Autodesk Inventor part; units mm, degrees
(part 6 of 7)
  line L4288 (-217.7033, 32.4949) -> (-217.7088, 32.0158)
  line L4289 (-217.7088, 32.0158) -> (-217.7607, 31.5383)
  line L4290 (-217.7607, 31.5383) -> (-217.8407, 31.2539)
  line L4291 (-217.8407, 31.2539) -> (-217.9599, 30.9836)
  line L4292 (-217.9599, 30.9836) -> (-218.06, 30.829)
  line L4293 (-218.06, 30.829) -> (-218.1762, 30.6868)
  line L4294 (-218.1762, 30.6868) -> (-218.3073, 30.5582)
  line L4295 (-218.3073, 30.5582) -> (-218.4521, 30.4446)
  line L4296 (-218.4521, 30.4446) -> (-218.6077, 30.3605)
  line L4297 (-218.6077, 30.3605) -> (-218.7713, 30.295)
  line L4298 (-218.7713, 30.295) -> (-218.9414, 30.2486)
  line L4299 (-218.9414, 30.2486) -> (-219.1162, 30.2219)
  line L4300 (-219.1162, 30.2219) -> (-219.7927, 30.1616)
  line L4301 (-219.7927, 30.1616) -> (-220.4717, 30.1477)
  line L4302 (-220.4717, 30.1477) -> (-225.6943, 30.1477)
  line L4303 (-225.6943, 30.1477) -> (-225.6943, 29.0188)
  line L4304 (-225.6943, 29.0188) -> (-226.8896, 29.0188)
  line L4305 (-226.8896, 29.0188) -> (-226.8896, 30.1477)
  line L4306 (-226.8896, 30.1477) -> (-229.1357, 30.1477)
  line L4307 (-229.1357, 30.1477) -> (-230.0615, 31.675)
  line L4308 (-230.0615, 31.675) -> (-226.8896, 31.675)
  line L4309 (-227.0654, -1.5867) -> (-226.9717, -1.1921)
  line L4310 (-226.9717, -1.1921) -> (-226.8154, -0.7976)
  line L4311 (-226.8154, -0.7976) -> (-226.6006, -0.3953)
  line L4312 (-226.6006, -0.3953) -> (-225.1709, -0.9265)
  line L4313 (-225.1709, -0.9265) -> (-225.3114, -1.1898)
  line L4314 (-225.3114, -1.1898) -> (-225.415, -1.4683)
  line L4315 (-225.415, -1.4683) -> (-225.4805, -1.7581)
  line L4316 (-225.4805, -1.7581) -> (-225.5068, -2.0554)
  line L4317 (-225.5068, -2.0554) -> (-225.4604, -2.423)
  line L4318 (-225.4604, -2.423) -> (-225.3285, -2.7636)
  line L4319 (-225.3285, -2.7636) -> (-225.1187, -3.0626)
  line L4320 (-225.1187, -3.0626) -> (-224.8389, -3.3054)
  line L4321 (-224.8389, -3.3054) -> (-224.6095, -3.4375)
  line L4322 (-224.6095, -3.4375) -> (-224.3623, -3.532)
  line L4323 (-224.3623, -3.532) -> (-223.9212, -3.6468)
  line L4324 (-223.9212, -3.6468) -> (-223.4735, -3.7282)
  line L4325 (-223.4735, -3.7282) -> (-223.0209, -3.7759)
  line L4326 (-223.0209, -3.7759) -> (-222.5654, -3.7898)
  line L4327 (-222.5654, -3.7898) -> (-217.8154, -3.7898)
  line L4328 (-217.8154, -3.7898) -> (-217.8154, -5.325)
  line L4329 (-217.8154, -5.325) -> (-226.8896, -5.325)
  line L4330 (-226.8896, -5.325) -> (-226.8896, -3.9421)
  line L4331 (-226.8896, -3.9421) -> (-225.5146, -3.9421)
  line L4332 (-225.5146, -3.9421) -> (-225.803, -3.7828)
  line L4333 (-225.803, -3.7828) -> (-226.0795, -3.6042)
  line L4334 (-226.0795, -3.6042) -> (-226.343, -3.4071)
  line L4335 (-226.343, -3.4071) -> (-226.5928, -3.1921)
  line L4336 (-226.5928, -3.1921) -> (-226.6972, -3.0847)
  line L4337 (-226.6972, -3.0847) -> (-226.7881, -2.9656)
  line L4338 (-226.7881, -2.9656) -> (-226.921, -2.7383)
  line L4339 (-226.921, -2.7383) -> (-227.0177, -2.495)
  line L4340 (-227.0177, -2.495) -> (-227.0767, -2.2399)
  line L4341 (-227.0767, -2.2399) -> (-227.0967, -1.9773)
  line L4342 (-227.0967, -1.9773) -> (-227.0654, -1.5867)
  line L4343 (-227.0654, 12.9368) -> (-226.9717, 13.3313)
  line L4344 (-226.9717, 13.3313) -> (-226.8154, 13.7297)
  line L4345 (-226.8154, 13.7297) -> (-226.6006, 14.1282)
  line L4346 (-226.6006, 14.1282) -> (-225.1709, 13.6008)
  line L4347 (-225.1709, 13.6008) -> (-225.3106, 13.3372)
  line L4348 (-225.3106, 13.3372) -> (-225.4139, 13.0587)
  line L4349 (-225.4139, 13.0587) -> (-225.4797, 12.769)
  line L4350 (-225.4797, 12.769) -> (-225.5068, 12.4719)
  line L4351 (-225.5068, 12.4719) -> (-225.4616, 12.1038)
  line L4352 (-225.4616, 12.1038) -> (-225.33, 11.763)
  line L4353 (-225.33, 11.763) -> (-225.1197, 11.464)
  line L4354 (-225.1197, 11.464) -> (-224.8389, 11.2219)
  line L4355 (-224.8389, 11.2219) -> (-224.6089, 11.0895)
  line L4356 (-224.6089, 11.0895) -> (-224.3623, 10.9914)
  line L4357 (-224.3623, 10.9914) -> (-223.9213, 10.877)
  line L4358 (-223.9213, 10.877) -> (-223.4735, 10.7964)
  line L4359 (-223.4735, 10.7964) -> (-223.0209, 10.7498)
  line L4360 (-223.0209, 10.7498) -> (-222.5654, 10.7375)
  line L4361 (-222.5654, 10.7375) -> (-217.8154, 10.7375)
  line L4362 (-217.8154, 10.7375) -> (-217.8154, 9.1985)
  line L4363 (-217.8154, 9.1985) -> (-226.8896, 9.1985)
  line L4364 (-226.8896, 9.1985) -> (-226.8896, 10.5813)
  line L4365 (-226.8896, 10.5813) -> (-225.5146, 10.5813)
  line L4366 (-225.5146, 10.5813) -> (-225.8025, 10.7415)
  line L4367 (-225.8025, 10.7415) -> (-226.0787, 10.9203)
  line L4368 (-226.0787, 10.9203) -> (-226.3424, 11.1171)
  line L4369 (-226.3424, 11.1171) -> (-226.5928, 11.3313)
  line L4370 (-226.5928, 11.3313) -> (-226.7777, 11.5469)
  line L4371 (-226.7777, 11.5469) -> (-226.9209, 11.7922)
  line L4372 (-226.9209, 11.7922) -> (-226.9978, 11.972)
  line L4373 (-226.9978, 11.972) -> (-227.0531, 12.1589)
  line L4374 (-227.0531, 12.1589) -> (-227.0862, 12.3509)
  line L4375 (-227.0862, 12.3509) -> (-227.0967, 12.5461)
  line L4376 (-227.0967, 12.5461) -> (-227.0654, 12.9368)
  line L4377 (-225.1982, -44.1804) -> (-225.1982, -37.6687)
  line L4378 (-225.1982, -37.6687) -> (-230.3428, -37.6687)
  line L4379 (-230.3428, -37.6687) -> (-230.3428, -36.0086)
  line L4380 (-230.3428, -36.0086) -> (-217.8154, -36.0086)
  line L4381 (-217.8154, -36.0086) -> (-217.8154, -37.6687)
  line L4382 (-217.8154, -37.6687) -> (-223.7217, -37.6687)
  line L4383 (-223.7217, -37.6687) -> (-223.7217, -44.1804)
  line L4384 (-223.7217, -44.1804) -> (-217.8154, -44.1804)
  line L4385 (-217.8154, -44.1804) -> (-217.8154, -45.8367)
  line L4386 (-217.8154, -45.8367) -> (-230.3428, -45.8367)
  line L4387 (-230.3428, -45.8367) -> (-230.3428, -44.1804)
  line L4388 (-230.3428, -44.1804) -> (-225.1982, -44.1804)
  line L4389 (-221.456, -21.0437) -> (-220.5474, -20.7358)
  line L4390 (-220.5474, -20.7358) -> (-219.6279, -20.4617)
  line L4391 (-219.6279, -20.4617) -> (-220.4966, -20.1929)
  line L4392 (-220.4966, -20.1929) -> (-221.3545, -19.8914)
  line L4393 (-221.3545, -19.8914) -> (-226.8896, -17.8757)
  line L4394 (-226.8896, -17.8757) -> (-226.8896, -16.2937)
  line L4395 (-226.8896, -16.2937) -> (-217.8154, -19.7273)
  line L4396 (-217.8154, -19.7273) -> (-217.8154, -21.1648)
  line L4397 (-217.8154, -21.1648) -> (-226.8896, -24.6179)
  line L4398 (-226.8896, -24.6179) -> (-226.8896, -22.9929)
  line L4399 (-226.8896, -22.9929) -> (-221.456, -21.0437)
  line L4400 (-230.5459, 28.0032) -> (-230.4917, 28.5563)
  line L4401 (-230.4917, 28.5563) -> (-230.4014, 29.1047)
  line L4402 (-230.4014, 29.1047) -> (-229.0615, 28.8743)
  line L4403 (-229.0615, 28.8743) -> (-229.1228, 28.4229)
  line L4404 (-229.1228, 28.4229) -> (-229.1474, 27.968)
  line L4405 (-229.1474, 27.968) -> (-229.1237, 27.6049)
  line L4406 (-229.1237, 27.6049) -> (-229.0303, 27.2532)
  line L4407 (-229.0303, 27.2532) -> (-228.9284, 27.0739)
  line L4408 (-228.9284, 27.0739) -> (-228.7871, 26.9279)
  line L4409 (-228.7871, 26.9279) -> (-228.6141, 26.8216)
  line L4410 (-228.6141, 26.8216) -> (-228.417, 26.761)
  line L4411 (-228.417, 26.761) -> (-228.0735, 26.7027)
  line L4412 (-228.0735, 26.7027) -> (-227.7256, 26.6868)
  line L4413 (-227.7256, 26.6868) -> (-226.8896, 26.6868)
  line L4414 (-226.8896, 26.6868) -> (-226.8896, 28.4563)
  line L4415 (-226.8896, 28.4563) -> (-225.6943, 28.4563)
  line L4416 (-225.6943, 28.4563) -> (-225.6943, 26.6868)
  line L4417 (-225.6943, 26.6868) -> (-217.8154, 26.6868)
  line L4418 (-217.8154, 26.6868) -> (-217.8154, 25.1594)
  line L4419 (-217.8154, 25.1594) -> (-225.6943, 25.1594)
  line L4420 (-225.6943, 25.1594) -> (-225.6943, 23.8)
  line L4421 (-225.6943, 23.8) -> (-226.8896, 23.8)
  line L4422 (-226.8896, 23.8) -> (-226.8896, 25.1594)
  line L4423 (-226.8896, 25.1594) -> (-227.5869, 25.157)
  line L4424 (-227.5869, 25.157) -> (-228.2842, 25.1672)
  line L4425 (-228.2842, 25.1672) -> (-228.6256, 25.1953)
  line L4426 (-228.6256, 25.1953) -> (-228.9639, 25.2493)
  line L4427 (-228.9639, 25.2493) -> (-229.2139, 25.3196)
  line L4428 (-229.2139, 25.3196) -> (-229.499, 25.4524)
  line L4429 (-229.499, 25.4524) -> (-229.7568, 25.6282)
  line L4430 (-229.7568, 25.6282) -> (-229.9834, 25.843)
  line L4431 (-229.9834, 25.843) -> (-230.1395, 26.0379)
  line L4432 (-230.1395, 26.0379) -> (-230.2724, 26.2493)
  line L4433 (-230.2724, 26.2493) -> (-230.3897, 26.5305)
  line L4434 (-230.3897, 26.5305) -> (-230.4754, 26.822)
  line L4435 (-230.4754, 26.822) -> (-230.529, 27.1211)
  line L4436 (-230.529, 27.1211) -> (-230.5498, 27.425)
  line L4437 (-230.5498, 27.425) -> (-230.5575, 27.7142)
  line L4438 (-230.5575, 27.7142) -> (-230.5459, 28.0032)
  line L4439 (-222.2842, 20.5618) -> (-222.123, 19.998)
  line L4440 (-222.123, 19.998) -> (-221.9865, 19.428)
  line L4441 (-221.9865, 19.428) -> (-221.8748, 18.8526)
  line L4442 (-221.8748, 18.8526) -> (-221.7881, 18.2727)
  line L4443 (-221.7881, 18.2727) -> (-221.6865, 17.6488)
  line L4444 (-221.6865, 17.6488) -> (-221.5224, 17.0383)
  line L4445 (-221.5224, 17.0383) -> (-221.4547, 16.8714)
  line L4446 (-221.4547, 16.8714) -> (-221.3669, 16.715)
  line L4447 (-221.3669, 16.715) -> (-221.2602, 16.5708)
  line L4448 (-221.2602, 16.5708) -> (-221.1357, 16.4407)
  line L4449 (-221.1357, 16.4407) -> (-220.9118, 16.2821)
  line L4450 (-220.9118, 16.2821) -> (-220.6683, 16.1747)
  line L4451 (-220.6683, 16.1747) -> (-220.4128, 16.1178)
  line L4452 (-220.4128, 16.1178) -> (-220.1531, 16.111)
  line L4453 (-220.1531, 16.111) -> (-219.8968, 16.1537)
  line L4454 (-219.8968, 16.1537) -> (-219.6517, 16.2453)
  line L4455 (-219.6517, 16.2453) -> (-219.4254, 16.3855)
  line L4456 (-219.4254, 16.3855) -> (-219.2256, 16.5735)
  line L4457 (-219.2256, 16.5735) -> (-219.101, 16.7434)
  line L4458 (-219.101, 16.7434) -> (-219.0001, 16.9273)
  line L4459 (-219.0001, 16.9273) -> (-218.9241, 17.1227)
  line L4460 (-218.9241, 17.1227) -> (-218.874, 17.3274)
  line L4461 (-218.874, 17.3274) -> (-218.8298, 17.6306)
  line L4462 (-218.8298, 17.6306) -> (-218.8154, 17.9368)
  line L4463 (-218.8154, 17.9368) -> (-218.8389, 18.3704)
  line L4464 (-218.8389, 18.3704) -> (-218.9131, 18.7766)
  line L4465 (-218.9131, 18.7766) -> (-219.0342, 19.1594)
  line L4466 (-219.0342, 19.1594) -> (-219.2021, 19.5188)
  line L4467 (-219.2021, 19.5188) -> (-219.417, 19.843)
  line L4468 (-219.417, 19.843) -> (-219.6631, 20.1204)
  line L4469 (-219.6631, 20.1204) -> (-219.9482, 20.3508)
  line L4470 (-219.9482, 20.3508) -> (-220.2685, 20.5344)
  line L4471 (-220.2685, 20.5344) -> (-220.5243, 20.6293)
  line L4472 (-220.5243, 20.6293) -> (-220.7871, 20.7002)
  line L4473 (-220.7871, 20.7002) -> (-221.0553, 20.7468)
  line L4474 (-221.0553, 20.7468) -> (-221.3271, 20.7688)
  line L4475 (-221.3271, 20.7688) -> (-221.8485, 20.7855)
  line L4476 (-221.8485, 20.7855) -> (-222.3701, 20.7844)
  line L4477 (-222.3701, 20.7844) -> (-222.2842, 20.5618)
  line L4478 (-225.8076, -30.0828) -> (-225.7184, -30.5473)
  line L4479 (-225.7184, -30.5473) -> (-225.5434, -30.982)
  line L4480 (-225.5434, -30.982) -> (-225.2885, -31.3754)
  line L4481 (-225.2885, -31.3754) -> (-224.9599, -31.7156)
  line L4482 (-224.9599, -31.7156) -> (-224.7132, -31.9024)
  line L4483 (-224.7132, -31.9024) -> (-224.4484, -32.0605)
  line L4484 (-224.4484, -32.0605) -> (-224.1678, -32.1888)
  line L4485 (-224.1678, -32.1888) -> (-223.874, -32.2859)
  line L4486 (-223.874, -32.2859) -> (-223.5001, -32.3748)
  line L4487 (-223.5001, -32.3748) -> (-223.1212, -32.4365)
  line L4488 (-223.1212, -32.4365) -> (-222.7388, -32.4707)
  line L4489 (-222.7388, -32.4707) -> (-222.3545, -32.4773)
  line L4490 (-222.3545, -32.4773) -> (-221.9682, -32.4706)
  line L4491 (-221.9682, -32.4706) -> (-221.5839, -32.4364)
  line L4492 (-221.5839, -32.4364) -> (-221.2031, -32.3748)
  line L4493 (-221.2031, -32.3748) -> (-220.8271, -32.2859)
  line L4494 (-220.8271, -32.2859) -> (-220.5333, -32.1888)
  line L4495 (-220.5333, -32.1888) -> (-220.2528, -32.0605)
  line L4496 (-220.2528, -32.0605) -> (-219.9879, -31.9024)
  line L4497 (-219.9879, -31.9024) -> (-219.7412, -31.7156)
  line L4498 (-219.7412, -31.7156) -> (-219.5426, -31.5267)
  line L4499 (-219.5426, -31.5267) -> (-219.3676, -31.319)
  line L4500 (-219.3676, -31.319) -> (-219.2175, -31.0945)
  line L4501 (-219.2175, -31.0945) -> (-219.0932, -30.8557)
  line L4502 (-219.0932, -30.8557) -> (-218.9956, -30.6047)
  line L4503 (-218.9956, -30.6047) -> (-218.9259, -30.3439)
  line L4504 (-218.9259, -30.3439) -> (-218.885, -30.0754)
  line L4505 (-218.885, -30.0754) -> (-218.874, -29.8015)
  line L4506 (-218.874, -29.8015) -> (-218.8857, -29.5284)
  line L4507 (-218.8857, -29.5284) -> (-218.9272, -29.2607)
  line L4508 (-218.9272, -29.2607) -> (-218.9975, -29.0007)
  line L4509 (-218.9975, -29.0007) -> (-219.0956, -28.7506)
  line L4510 (-219.0956, -28.7506) -> (-219.2205, -28.5128)
  line L4511 (-219.2205, -28.5128) -> (-219.371, -28.2895)
  line L4512 (-219.371, -28.2895) -> (-219.5462, -28.0829)
  line L4513 (-219.5462, -28.0829) -> (-219.7451, -27.8953)
  line L4514 (-219.7451, -27.8953) -> (-219.9964, -27.7091)
  line L4515 (-219.9964, -27.7091) -> (-220.2654, -27.5512)
  line L4516 (-220.2654, -27.5512) -> (-220.5496, -27.4227)
  line L4517 (-220.5496, -27.4227) -> (-220.8467, -27.325)
  line L4518 (-220.8467, -27.325) -> (-221.5172, -27.1955)
  line L4519 (-221.5172, -27.1955) -> (-222.1958, -27.1386)
  line L4520 (-222.1958, -27.1386) -> (-222.8765, -27.1544)
  line L4521 (-222.8765, -27.1544) -> (-223.5537, -27.2429)
  line L4522 (-223.5537, -27.2429) -> (-223.8631, -27.3185)
  line L4523 (-223.8631, -27.3185) -> (-224.163, -27.4237)
  line L4524 (-224.163, -27.4237) -> (-224.4512, -27.5577)
  line L4525 (-224.4512, -27.5577) -> (-224.7256, -27.7195)
  line L4526 (-224.7256, -27.7195) -> (-224.9961, -27.9333)
  line L4527 (-224.9961, -27.9333) -> (-225.2347, -28.18)
  line L4528 (-225.2347, -28.18) -> (-225.4385, -28.4563)
  line L4529 (-225.4385, -28.4563) -> (-225.6045, -28.7586)
  line L4530 (-225.6045, -28.7586) -> (-225.7202, -29.0775)
  line L4531 (-225.7202, -29.0775) -> (-225.7931, -29.4073)
  line L4532 (-225.7931, -29.4073) -> (-225.8225, -29.7438)
  line L4533 (-225.8225, -29.7438) -> (-225.8076, -30.0828)
  line L4534 (-225.8193, -11.6257) -> (-225.7669, -11.9667)
  line L4535 (-225.7669, -11.9667) -> (-225.6692, -12.2923)
  line L4536 (-225.6692, -12.2923) -> (-225.5291, -12.5988)
  line L4537 (-225.5291, -12.5988) -> (-225.3494, -12.8822)
  line L4538 (-225.3494, -12.8822) -> (-225.133, -13.1387)
  line L4539 (-225.133, -13.1387) -> (-224.8827, -13.3644)
  line L4540 (-224.8827, -13.3644) -> (-224.6014, -13.5554)
  line L4541 (-224.6014, -13.5554) -> (-224.292, -13.7078)
  line L4542 (-224.292, -13.7078) -> (-224.0337, -13.8014)
  line L4543 (-224.0337, -13.8014) -> (-223.769, -13.8725)
  line L4544 (-223.769, -13.8725) -> (-223.4991, -13.9208)
  line L4545 (-223.4991, -13.9208) -> (-223.2256, -13.9461)
  line L4546 (-223.2256, -13.9461) -> (-223.2256, -8.8796)
  line L4547 (-223.2256, -8.8796) -> (-223.5351, -8.9115)
  line L4548 (-223.5351, -8.9115) -> (-223.8405, -8.9686)
  line L4549 (-223.8405, -8.9686) -> (-224.1402, -9.0505)
  line L4550 (-224.1402, -9.0505) -> (-224.4326, -9.157)
  line L4551 (-224.4326, -9.157) -> (-224.7123, -9.303)
  line L4552 (-224.7123, -9.303) -> (-224.9664, -9.4829)
  line L4553 (-224.9664, -9.4829) -> (-225.1923, -9.6932)
  line L4554 (-225.1923, -9.6932) -> (-225.3877, -9.9305)
  line L4555 (-225.3877, -9.9305) -> (-225.5502, -10.1915)
  line L4556 (-225.5502, -10.1915) -> (-225.6772, -10.4728)
  line L4557 (-225.6772, -10.4728) -> (-225.7664, -10.771)
  line L4558 (-225.7664, -10.771) -> (-225.8154, -11.0828)
  line L4559 (-225.8154, -11.0828) -> (-225.831, -11.3542)
  line L4560 (-225.831, -11.3542) -> (-225.8193, -11.6257)
  line L4561 (-247.2099, -34.1531) -> (-247.1518, -33.6767)
  line L4562 (-247.1518, -33.6767) -> (-247.0312, -33.219)
  line L4563 (-247.0312, -33.219) -> (-246.8517, -32.7853)
  line L4564 (-246.8517, -32.7853) -> (-246.617, -32.381)
  line L4565 (-246.617, -32.381) -> (-246.3307, -32.0114)
  line L4566 (-246.3307, -32.0114) -> (-245.9964, -31.6819)
  line L4567 (-245.9964, -31.6819) -> (-245.6177, -31.3979)
  line L4568 (-245.6177, -31.3979) -> (-245.1982, -31.1648)
  line L4569 (-245.1982, -31.1648) -> (-244.9326, -31.0476)
  line L4570 (-244.9326, -31.0476) -> (-244.3779, -30.8484)
  line L4571 (-244.3779, -30.8484) -> (-243.792, -30.7078)
  line L4572 (-243.792, -30.7078) -> (-243.1826, -30.6218)
  line L4573 (-243.1826, -30.6218) -> (-242.5459, -30.5945)
  line L4574 (-242.5459, -30.5945) -> (-241.9016, -30.6187)
  line L4575 (-241.9016, -30.6187) -> (-241.2653, -30.7109)
  line L4576 (-241.2653, -30.7109) -> (-240.6424, -30.8698)
  line L4577 (-240.6424, -30.8698) -> (-240.0381, -31.0945)
  line L4578 (-240.0381, -31.0945) -> (-239.593, -31.3209)
  line L4579 (-239.593, -31.3209) -> (-239.1828, -31.6022)
  line L4580 (-239.1828, -31.6022) -> (-238.8125, -31.9343)
  line L4581 (-238.8125, -31.9343) -> (-238.4873, -32.3132)
  line L4582 (-238.4873, -32.3132) -> (-238.1679, -32.8229)
  line L4583 (-238.1679, -32.8229) -> (-237.9334, -33.3728)
  line L4584 (-237.9334, -33.3728) -> (-237.7874, -33.9525)
  line L4585 (-237.7874, -33.9525) -> (-237.7334, -34.5515)
  line L4586 (-237.7334, -34.5515) -> (-237.7557, -34.9169)
  line L4587 (-237.7557, -34.9169) -> (-237.8154, -35.2781)
  line L4588 (-237.8154, -35.2781) -> (-237.9778, -35.7534)
  line L4589 (-237.9778, -35.7534) -> (-238.2133, -36.1934)
  line L4590 (-238.2133, -36.1934) -> (-238.5164, -36.5898)
  line L4591 (-238.5164, -36.5898) -> (-238.8818, -36.9343)
  line L4592 (-238.8818, -36.9343) -> (-234.4639, -36.9343)
  line L4593 (-234.4639, -36.9343) -> (-234.4639, -38.4734)
  line L4594 (-234.4639, -38.4734) -> (-247.0146, -38.4734)
  line L4595 (-247.0146, -38.4734) -> (-247.0146, -37.0711)
  line L4596 (-247.0146, -37.0711) -> (-245.8349, -37.0711)
  line L4597 (-245.8349, -37.0711) -> (-246.1499, -36.8214)
  line L4598 (-246.1499, -36.8214) -> (-246.4404, -36.5437)
  line L4599 (-246.4404, -36.5437) -> (-246.6749, -36.2598)
  line L4600 (-246.6749, -36.2598) -> (-246.874, -35.95)
  line L4601 (-246.874, -35.95) -> (-247.0264, -35.6218)
  line L4602 (-247.0264, -35.6218) -> (-247.1347, -35.25)
  line L4603 (-247.1347, -35.25) -> (-247.1982, -34.8679)
  line L4604 (-247.1982, -34.8679) -> (-247.2212, -34.5108)
  line L4605 (-247.2212, -34.5108) -> (-247.2099, -34.1531)
  line L4606 (-247.2021, -20.6804) -> (-247.1633, -20.3627)
  line L4607 (-247.1633, -20.3627) -> (-247.1019, -20.049)
  line L4608 (-247.1019, -20.049) -> (-247.0185, -19.7405)
  line L4609 (-247.0185, -19.7405) -> (-246.9131, -19.4382)
  line L4610 (-246.9131, -19.4382) -> (-246.7876, -19.1567)
  line L4611 (-246.7876, -19.1567) -> (-246.6398, -18.8869)
  line L4612 (-246.6398, -18.8869) -> (-246.4704, -18.63)
  line L4613 (-246.4704, -18.63) -> (-246.2803, -18.3875)
  line L4614 (-246.2803, -18.3875) -> (-245.9951, -18.0789)
  line L4615 (-245.9951, -18.0789) -> (-245.672, -17.8024)
  line L4616 (-245.672, -17.8024) -> (-245.3232, -17.5593)
  line L4617 (-245.3232, -17.5593) -> (-245.0317, -17.3993)
  line L4618 (-245.0317, -17.3993) -> (-244.7292, -17.2622)
  line L4619 (-244.7292, -17.2622) -> (-244.417, -17.1487)
  line L4620 (-244.417, -17.1487) -> (-244.0967, -17.0593)
  line L4621 (-244.0967, -17.0593) -> (-243.7278, -16.9846)
  line L4622 (-243.7278, -16.9846) -> (-243.3555, -16.9316)
  line L4623 (-243.3555, -16.9316) -> (-242.9807, -16.9005)
  line L4624 (-242.9807, -16.9005) -> (-242.6045, -16.8914)
  line L4625 (-242.6045, -16.8914) -> (-241.8202, -16.9221)
  line L4626 (-241.8202, -16.9221) -> (-241.042, -17.0242)
  line L4627 (-241.042, -17.0242) -> (-240.6648, -17.1051)
  line L4628 (-240.6648, -17.1051) -> (-240.2979, -17.2212)
  line L4629 (-240.2979, -17.2212) -> (-239.9436, -17.3717)
  line L4630 (-239.9436, -17.3717) -> (-239.6045, -17.5554)
  line L4631 (-239.6045, -17.5554) -> (-239.3457, -17.7346)
  line L4632 (-239.3457, -17.7346) -> (-239.1032, -17.933)
  line L4633 (-239.1032, -17.933) -> (-238.8781, -18.1494)
  line L4634 (-238.8781, -18.1494) -> (-238.6713, -18.3827)
  line L4635 (-238.6713, -18.3827) -> (-238.4837, -18.6318)
  line L4636 (-238.4837, -18.6318) -> (-238.3163, -18.8954)
  line L4637 (-238.3163, -18.8954) -> (-238.1701, -19.1724)
  line L4638 (-238.1701, -19.1724) -> (-238.0459, -19.4617)
  line L4639 (-238.0459, -19.4617) -> (-237.9085, -19.8681)
  line L4640 (-237.9085, -19.8681) -> (-237.8103, -20.2848)
  line L4641 (-237.8103, -20.2848) -> (-237.7517, -20.7088)
  line L4642 (-237.7517, -20.7088) -> (-237.7334, -21.1375)
  line L4643 (-237.7334, -21.1375) -> (-237.7427, -21.4733)
  line L4644 (-237.7427, -21.4733) -> (-237.7745, -21.8073)
  line L4645 (-237.7745, -21.8073) -> (-237.8287, -22.1385)
  line L4646 (-237.8287, -22.1385) -> (-237.9053, -22.4656)
  line L4647 (-237.9053, -22.4656) -> (-238.0021, -22.7599)
  line L4648 (-238.0021, -22.7599) -> (-238.1207, -23.0456)
  line L4649 (-238.1207, -23.0456) -> (-238.2604, -23.3216)
  line L4650 (-238.2604, -23.3216) -> (-238.4209, -23.5867)
  line L4651 (-238.4209, -23.5867) -> (-238.6077, -23.8396)
  line L4652 (-238.6077, -23.8396) -> (-238.814, -24.0763)
  line L4653 (-238.814, -24.0763) -> (-239.0385, -24.2958)
  line L4654 (-239.0385, -24.2958) -> (-239.2803, -24.4968)
  line L4655 (-239.2803, -24.4968) -> (-239.6357, -24.7351)
  line L4656 (-239.6357, -24.7351) -> (-239.9386, -24.8944)
  line L4657 (-239.9386, -24.8944) -> (-240.252, -25.0305)
  line L4658 (-240.252, -25.0305) -> (-240.5747, -25.143)
  line L4659 (-240.5747, -25.143) -> (-240.9053, -25.2312)
  line L4660 (-240.9053, -25.2312) -> (-241.2951, -25.3039)
  line L4661 (-241.2951, -25.3039) -> (-241.688, -25.3555)
  line L4662 (-241.688, -25.3555) -> (-242.083, -25.386)
  line L4663 (-242.083, -25.386) -> (-242.4795, -25.3953)
  line L4664 (-242.4795, -25.3953) -> (-243.0691, -25.3734)
  line L4665 (-243.0691, -25.3734) -> (-243.6553, -25.3054)
  line L4666 (-243.6553, -25.3054) -> (-244.1826, -25.1961)
  line L4667 (-244.1826, -25.1961) -> (-244.6709, -25.0437)
  line L4668 (-244.6709, -25.0437) -> (-245.1162, -24.8484)
  line L4669 (-245.1162, -24.8484) -> (-245.5224, -24.6062)
  line L4670 (-245.5224, -24.6062) -> (-245.8896, -24.3211)
  line L4671 (-245.8896, -24.3211) -> (-246.2139, -23.9929)
  line L4672 (-246.2139, -23.9929) -> (-246.5557, -23.5359)
  line L4673 (-246.5557, -23.5359) -> (-246.8289, -23.0379)
  line L4674 (-246.8289, -23.0379) -> (-247.0299, -22.5067)
  line L4675 (-247.0299, -22.5067) -> (-247.1553, -21.95)
  line L4676 (-247.1553, -21.95) -> (-247.1969, -21.6341)
  line L4677 (-247.1969, -21.6341) -> (-247.2186, -21.3167)
  line L4678 (-247.2186, -21.3167) -> (-247.2203, -20.9984)
  line L4679 (-247.2203, -20.9984) -> (-247.2021, -20.6804)
  line L4680 (-245.999, 16.7805) -> (-246.2791, 17.0294)
  line L4681 (-246.2791, 17.0294) -> (-246.5342, 17.3039)
  line L4682 (-246.5342, 17.3039) -> (-246.7411, 17.5857)
  line L4683 (-246.7411, 17.5857) -> (-246.9127, 17.8888)
  line L4684 (-246.9127, 17.8888) -> (-247.0474, 18.2101)
  line L4685 (-247.0474, 18.2101) -> (-247.1435, 18.5461)
  line L4686 (-247.1435, 18.5461) -> (-247.203, 18.9053)
  line L4687 (-247.203, 18.9053) -> (-247.2217, 19.2688)
  line L4688 (-247.2217, 19.2688) -> (-247.2097, 19.5755)
  line L4689 (-247.2097, 19.5755) -> (-247.1736, 19.8799)
  line L4690 (-247.1736, 19.8799) -> (-247.1138, 20.1804)
  line L4691 (-247.1138, 20.1804) -> (-247.0303, 20.4758)
  line L4692 (-247.0303, 20.4758) -> (-246.8832, 20.8516)
  line L4693 (-246.8832, 20.8516) -> (-246.6982, 21.2102)
  line L4694 (-246.6982, 21.2102) -> (-246.4773, 21.5322)
  line L4695 (-246.4773, 21.5322) -> (-246.2217, 21.8274)
  line L4696 (-246.2217, 21.8274) -> (-246.0013, 22.0259)
  line L4697 (-246.0013, 22.0259) -> (-245.767, 22.2071)
  line L4698 (-245.767, 22.2071) -> (-245.5198, 22.3704)
  line L4699 (-245.5198, 22.3704) -> (-245.2607, 22.5149)
  line L4700 (-245.2607, 22.5149) -> (-244.7435, 22.7407)
  line L4701 (-244.7435, 22.7407) -> (-244.2077, 22.9137)
  line L4702 (-244.2077, 22.9137) -> (-243.6574, 23.0328)
  line L4703 (-243.6574, 23.0328) -> (-243.0967, 23.0969)
  line L4704 (-243.0967, 23.0969) -> (-242.7005, 23.1132)
  line L4705 (-242.7005, 23.1132) -> (-242.3043, 23.1095)
  line L4706 (-242.3043, 23.1095) -> (-241.9087, 23.0859)
  line L4707 (-241.9087, 23.0859) -> (-241.5146, 23.0422)
  line L4708 (-241.5146, 23.0422) -> (-241.0258, 22.9549)
  line L4709 (-241.0258, 22.9549) -> (-240.5459, 22.8274)
  line L4710 (-240.5459, 22.8274) -> (-240.119, 22.6663)
  line L4711 (-240.119, 22.6663) -> (-239.7099, 22.4641)
  line L4712 (-239.7099, 22.4641) -> (-239.275, 22.1779)
  line L4713 (-239.275, 22.1779) -> (-238.881, 21.8407)
  line L4714 (-238.881, 21.8407) -> (-238.5323, 21.4568)
  line L4715 (-238.5323, 21.4568) -> (-238.2334, 21.0305)
  line L4716 (-238.2334, 21.0305) -> (-238.0531, 20.6923)
  line L4717 (-238.0531, 20.6923) -> (-237.9128, 20.337)
  line L4718 (-237.9128, 20.337) -> (-237.8137, 19.9681)
  line L4719 (-237.8137, 19.9681) -> (-237.7568, 19.5891)
  line L4720 (-237.7568, 19.5891) -> (-237.7356, 19.2988)
  line L4721 (-237.7356, 19.2988) -> (-237.7391, 19.0083)
  line L4722 (-237.7391, 19.0083) -> (-237.767, 18.7192)
  line L4723 (-237.767, 18.7192) -> (-237.8193, 18.4329)
  line L4724 (-237.8193, 18.4329) -> (-237.924, 18.0874)
  line L4725 (-237.924, 18.0874) -> (-238.0693, 17.7571)
  line L4726 (-238.0693, 17.7571) -> (-238.2708, 17.4415)
  line L4727 (-238.2708, 17.4415) -> (-238.5077, 17.1533)
  line L4728 (-238.5077, 17.1533) -> (-238.7774, 16.8955)
  line L4729 (-238.7774, 16.8955) -> (-239.0771, 16.6711)
  line L4730 (-239.0771, 16.6711) -> (-237.9404, 16.6711)
  line L4731 (-237.9404, 16.6711) -> (-237.9404, 15.2454)
  line L4732 (-237.9404, 15.2454) -> (-250.4678, 15.2454)
  line L4733 (-250.4678, 15.2454) -> (-250.4678, 16.7805)
  line L4734 (-250.4678, 16.7805) -> (-245.999, 16.7805)
  line L4735 (-247.2178, 3.8) -> (-247.1979, 4.2075)
  line L4736 (-247.1979, 4.2075) -> (-247.1461, 4.6114)
  line L4737 (-247.1461, 4.6114) -> (-247.0628, 5.0101)
  line L4738 (-247.0628, 5.0101) -> (-246.9482, 5.4016)
  line L4739 (-246.9482, 5.4016) -> (-246.8079, 5.7248)
  line L4740 (-246.8079, 5.7248) -> (-246.6396, 6.0344)
  line L4741 (-246.6396, 6.0344) -> (-246.4652, 6.2661)
  line L4742 (-246.4652, 6.2661) -> (-246.2607, 6.4719)
  line L4743 (-246.2607, 6.4719) -> (-245.8968, 6.7018)
  line L4744 (-245.8968, 6.7018) -> (-245.5033, 6.8694)
  line L4745 (-245.5033, 6.8694) -> (-245.0882, 6.972)
  line L4746 (-245.0882, 6.972) -> (-244.6592, 7.0071)
  line L4747 (-244.6592, 7.0071) -> (-244.3507, 7.0202)
  line L4748 (-244.3507, 7.0202) -> (-244.042, 7.0266)
  line L4749 (-244.042, 7.0266) -> (-241.2295, 7.0266)
  line L4750 (-241.2295, 7.0266) -> (-240.3208, 7.039)
  line L4751 (-240.3208, 7.039) -> (-239.4131, 7.0813)
  line L4752 (-239.4131, 7.0813) -> (-239.0281, 7.1259)
  line L4753 (-239.0281, 7.1259) -> (-238.6519, 7.2137)
  line L4754 (-238.6519, 7.2137) -> (-238.2881, 7.3438)
  line L4755 (-238.2881, 7.3438) -> (-237.9404, 7.5149)
  line L4756 (-237.9404, 7.5149) -> (-237.9404, 5.9055)
  line L4757 (-237.9404, 5.9055) -> (-238.2096, 5.7919)
  line L4758 (-238.2096, 5.7919) -> (-238.4873, 5.7029)
  line L4759 (-238.4873, 5.7029) -> (-238.7718, 5.6391)
  line L4760 (-238.7718, 5.6391) -> (-239.0615, 5.6008)
  line L4761 (-239.0615, 5.6008) -> (-238.7348, 5.1928)
  line L4762 (-238.7348, 5.1928) -> (-238.4404, 4.761)
  line L4763 (-238.4404, 4.761) -> (-238.217, 4.3689)
  line L4764 (-238.217, 4.3689) -> (-238.0342, 3.9563)
  line L4765 (-238.0342, 3.9563) -> (-237.8425, 3.2909)
  line L4766 (-237.8425, 3.2909) -> (-237.7455, 2.6087)
  line L4767 (-237.7455, 2.6087) -> (-237.7441, 1.9196)
  line L4768 (-237.7441, 1.9196) -> (-237.8389, 1.2336)
  line L4769 (-237.8389, 1.2336) -> (-237.9123, 0.9517)
  line L4770 (-237.9123, 0.9517) -> (-238.0136, 0.6792)
  line L4771 (-238.0136, 0.6792) -> (-238.1417, 0.4184)
  line L4772 (-238.1417, 0.4184) -> (-238.2959, 0.1711)
  line L4773 (-238.2959, 0.1711) -> (-238.4854, -0.0613)
  line L4774 (-238.4854, -0.0613) -> (-238.6995, -0.2665)
  line L4775 (-238.6995, -0.2665) -> (-238.9352, -0.443)
  line L4776 (-238.9352, -0.443) -> (-239.1895, -0.5894)
  line L4777 (-239.1895, -0.5894) -> (-239.4596, -0.7042)
  line L4778 (-239.4596, -0.7042) -> (-239.7425, -0.786)
  line L4779 (-239.7425, -0.786) -> (-240.0353, -0.8332)
  line L4780 (-240.0353, -0.8332) -> (-240.3349, -0.8445)
  line L4781 (-240.3349, -0.8445) -> (-240.6848, -0.8207)
  line L4782 (-240.6848, -0.8207) -> (-241.0235, -0.7506)
  line L4783 (-241.0235, -0.7506) -> (-241.3468, -0.6366)
  line L4784 (-241.3468, -0.6366) -> (-241.6509, -0.4811)
  line L4785 (-241.6509, -0.4811) -> (-241.9315, -0.2866)
  line L4786 (-241.9315, -0.2866) -> (-242.1848, -0.0555)
  line L4787 (-242.1848, -0.0555) -> (-242.4065, 0.2099)
  line L4788 (-242.4065, 0.2099) -> (-242.5928, 0.5071)
  line L4789 (-242.5928, 0.5071) -> (-242.7571, 0.8456)
  line L4790 (-242.7571, 0.8456) -> (-242.8898, 1.1969)
  line L4791 (-242.8898, 1.1969) -> (-242.9902, 1.5587)
  line L4792 (-242.9902, 1.5587) -> (-243.0576, 1.9289)
  line L4793 (-243.0576, 1.9289) -> (-243.1964, 2.9591)
  line L4794 (-243.1964, 2.9591) -> (-243.3467, 3.9875)
  line L4795 (-243.3467, 3.9875) -> (-243.4927, 4.7368)
  line L4796 (-243.4927, 4.7368) -> (-243.6982, 5.4719)
  line L4797 (-243.6982, 5.4719) -> (-244.2155, 5.4752)
  line L4798 (-244.2155, 5.4752) -> (-244.7295, 5.4172)
  line L4799 (-244.7295, 5.4172) -> (-245.0399, 5.3163)
  line L4800 (-245.0399, 5.3163) -> (-245.3193, 5.1477)
  line L4801 (-245.3193, 5.1477) -> (-245.4869, 4.9667)
  line L4802 (-245.4869, 4.9667) -> (-245.6267, 4.7649)
  line L4803 (-245.6267, 4.7649) -> (-245.7368, 4.5456)
  line L4804 (-245.7368, 4.5456) -> (-245.8154, 4.3118)
  line L4805 (-245.8154, 4.3118) -> (-245.8873, 3.9963)
  line L4806 (-245.8873, 3.9963) -> (-245.9322, 3.6764)
  line L4807 (-245.9322, 3.6764) -> (-245.9499, 3.3539)
  line L4808 (-245.9499, 3.3539) -> (-245.9404, 3.0305)
  line L4809 (-245.9404, 3.0305) -> (-245.9212, 2.7189)
  line L4810 (-245.9212, 2.7189) -> (-245.8668, 2.4126)
  line L4811 (-245.8668, 2.4126) -> (-245.7779, 2.1144)
  line L4812 (-245.7779, 2.1144) -> (-245.6553, 1.8274)
  line L4813 (-245.6553, 1.8274) -> (-245.5327, 1.6508)
  line L4814 (-245.5327, 1.6508) -> (-245.3882, 1.493)
  line L4815 (-245.3882, 1.493) -> (-245.224, 1.3558)
  line L4816 (-245.224, 1.3558) -> (-245.042, 1.2414)
  line L4817 (-245.042, 1.2414) -> (-244.6423, 1.056)
  line L4818 (-244.6423, 1.056) -> (-244.2217, 0.925)
  line L4819 (-244.2217, 0.925) -> (-244.4248, -0.5789)
  line L4820 (-244.4248, -0.5789) -> (-244.8688, -0.4631)
  line L4821 (-244.8688, -0.4631) -> (-245.2998, -0.3054)
  line L4822 (-245.2998, -0.3054) -> (-245.667, -0.1218)
  line L4823 (-245.667, -0.1218) -> (-245.9873, 0.0969)
  line L4824 (-245.9873, 0.0969) -> (-246.2468, 0.3426)
  line L4825 (-246.2468, 0.3426) -> (-246.4729, 0.6174)
  line L4826 (-246.4729, 0.6174) -> (-246.6632, 0.9182)
  line L4827 (-246.6632, 0.9182) -> (-246.8154, 1.2414)
  line L4828 (-246.8154, 1.2414) -> (-246.9014, 1.4563)
  line L4829 (-246.9014, 1.4563) -> (-247.0412, 1.9297)
  line L4830 (-247.0412, 1.9297) -> (-247.1396, 2.4133)
  line L4831 (-247.1396, 2.4133) -> (-247.2091, 3.105)
  line L4832 (-247.2091, 3.105) -> (-247.2178, 3.8)
  line L4833 (-247.2021, 29.2219) -> (-247.1477, 29.631)
  line L4834 (-247.1477, 29.631) -> (-247.0514, 30.0313)
  line L4835 (-247.0514, 30.0313) -> (-246.9143, 30.4194)
  line L4836 (-246.9143, 30.4194) -> (-246.7373, 30.7922)
  line L4837 (-246.7373, 30.7922) -> (-246.5718, 31.0616)
  line L4838 (-246.5718, 31.0616) -> (-246.3861, 31.3155)
  line L4839 (-246.3861, 31.3155) -> (-246.1812, 31.5528)
  line L4840 (-246.1812, 31.5528) -> (-245.9583, 31.7727)
  line L4841 (-245.9583, 31.7727) -> (-245.7186, 31.974)
  line L4842 (-245.7186, 31.974) -> (-245.463, 32.1557)
  line L4843 (-245.463, 32.1557) -> (-245.1928, 32.3168)
  line L4844 (-245.1928, 32.3168) -> (-244.9092, 32.4563)
  line L4845 (-244.9092, 32.4563) -> (-244.4805, 32.62)
  line L4846 (-244.4805, 32.62) -> (-244.0381, 32.7414)
  line L4847 (-244.0381, 32.7414) -> (-243.5434, 32.8367)
  line L4848 (-243.5434, 32.8367) -> (-243.042, 32.886)
  line L4849 (-243.042, 32.886) -> (-242.7296, 32.9013)
  line L4850 (-242.7296, 32.9013) -> (-242.417, 32.9055)
  line L4851 (-242.417, 32.9055) -> (-242.2509, 32.9021)
  line L4852 (-242.2509, 32.9021) -> (-242.0849, 32.8977)
  line L4853 (-242.0849, 32.8977) -> (-242.0849, 26.1282)
  line L4854 (-242.0849, 26.1282) -> (-241.7487, 26.1561)
  line L4855 (-241.7487, 26.1561) -> (-241.4157, 26.2079)
  line L4856 (-241.4157, 26.2079) -> (-241.0873, 26.2833)
  line L4857 (-241.0873, 26.2833) -> (-240.7646, 26.3821)
  line L4858 (-240.7646, 26.3821) -> (-240.3232, 26.5832)
  line L4859 (-240.3232, 26.5832) -> (-239.9279, 26.8577)
  line L4860 (-239.9279, 26.8577) -> (-239.5877, 27.1981)
  line L4861 (-239.5877, 27.1981) -> (-239.3115, 27.5969)
  line L4862 (-239.3115, 27.5969) -> (-239.1803, 27.8836)
  line L4863 (-239.1803, 27.8836) -> (-239.0841, 28.1805)
  line L4864 (-239.0841, 28.1805) -> (-239.0232, 28.4846)
  line L4865 (-239.0232, 28.4846) -> (-238.9975, 28.7927)
  line L4866 (-238.9975, 28.7927) -> (-239.0072, 29.1017)
  line L4867 (-239.0072, 29.1017) -> (-239.0522, 29.4085)
  line L4868 (-239.0522, 29.4085) -> (-239.1328, 29.71)
  line L4869 (-239.1328, 29.71) -> (-239.249, 30.0032)
  line L4870 (-239.249, 30.0032) -> (-239.3983, 30.2526)
  line L4871 (-239.3983, 30.2526) -> (-239.5788, 30.479)
  line L4872 (-239.5788, 30.479) -> (-239.7877, 30.6793)
  line L4873 (-239.7877, 30.6793) -> (-240.0224, 30.8508)
  line L4874 (-240.0224, 30.8508) -> (-240.4294, 31.0842)
  line L4875 (-240.4294, 31.0842) -> (-240.8623, 31.2649)
  line L4876 (-240.8623, 31.2649) -> (-240.667, 32.8547)
  line L4877 (-240.667, 32.8547) -> (-240.2666, 32.7316)
  line L4878 (-240.2666, 32.7316) -> (-239.8812, 32.5699)
  line L4879 (-239.8812, 32.5699) -> (-239.5138, 32.3709)
  line L4880 (-239.5138, 32.3709) -> (-239.167, 32.136)
  line L4881 (-239.167, 32.136) -> (-238.7507, 31.7564)
  line L4882 (-238.7507, 31.7564) -> (-238.4017, 31.3187)
  line L4883 (-238.4017, 31.3187) -> (-238.1257, 30.8317)
  line L4884 (-238.1257, 30.8317) -> (-237.9287, 30.3039)
  line L4885 (-237.9287, 30.3039) -> (-237.8417, 29.9495)
  line L4886 (-237.8417, 29.9495) -> (-237.78, 29.5902)
  line L4887 (-237.78, 29.5902) -> (-237.7439, 29.2274)
  line L4888 (-237.7439, 29.2274) -> (-237.7334, 28.8625)
  line L4889 (-237.7334, 28.8625) -> (-237.7519, 28.3901)
  line L4890 (-237.7519, 28.3901) -> (-237.8115, 27.9211)
  line L4891 (-237.8115, 27.9211) -> (-237.9074, 27.494)
  line L4892 (-237.9074, 27.494) -> (-238.042, 27.0774)
  line L4893 (-238.042, 27.0774) -> (-238.2645, 26.6044)
  line L4894 (-238.2645, 26.6044) -> (-238.5487, 26.1687)
  line L4895 (-238.5487, 26.1687) -> (-238.8901, 25.7762)
  line L4896 (-238.8901, 25.7762) -> (-239.2842, 25.4329)
  line L4897 (-239.2842, 25.4329) -> (-239.6357, 25.1946)
  line L4898 (-239.6357, 25.1946) -> (-239.9321, 25.0375)
  line L4899 (-239.9321, 25.0375) -> (-240.2387, 24.9028)
  line L4900 (-240.2387, 24.9028) -> (-240.5544, 24.7909)
  line L4901 (-240.5544, 24.7909) -> (-240.8779, 24.7024)
  line L4902 (-240.8779, 24.7024) -> (-241.2549, 24.6298)
  line L4903 (-241.2549, 24.6298) -> (-241.6351, 24.5782)
  line L4904 (-241.6351, 24.5782) -> (-242.0175, 24.5477)
  line L4905 (-242.0175, 24.5477) -> (-242.4014, 24.5383)
  line L4906 (-242.4014, 24.5383) -> (-242.9436, 24.557)
  line L4907 (-242.9436, 24.557) -> (-243.4834, 24.6125)
  line L4908 (-243.4834, 24.6125) -> (-243.9646, 24.7037)
  line L4909 (-243.9646, 24.7037) -> (-244.4365, 24.8352)
  line L4910 (-244.4365, 24.8352) -> (-244.8581, 24.9974)
  line L4911 (-244.8581, 24.9974) -> (-245.2607, 25.2024)
  line L4912 (-245.2607, 25.2024) -> (-245.6214, 25.4426)
  line L4913 (-245.6214, 25.4426) -> (-245.956, 25.718)
  line L4914 (-245.956, 25.718) -> (-246.2483, 26.0213)
  line L4915 (-246.2483, 26.0213) -> (-246.5107, 26.3508)
  line L4916 (-246.5107, 26.3508) -> (-246.7256, 26.7025)
  line L4917 (-246.7256, 26.7025) -> (-246.9053, 27.0735)
  line L4918 (-246.9053, 27.0735) -> (-247.0454, 27.4864)
  line L4919 (-247.0454, 27.4864) -> (-247.1452, 27.9098)
  line L4920 (-247.1452, 27.9098) -> (-247.2041, 28.3409)
  line L4921 (-247.2041, 28.3409) -> (-247.2217, 28.7766)
  line L4922 (-247.2217, 28.7766) -> (-247.2021, 29.2219)
  line L4923 (-247.0146, 40.5149) -> (-247.0146, 42.0618)
  line L4924 (-247.0146, 42.0618) -> (-245.8193, 42.0618)
  line L4925 (-245.8193, 42.0618) -> (-245.8193, 40.5149)
  line L4926 (-245.8193, 40.5149) -> (-240.5107, 40.5149)
  line L4927 (-240.5107, 40.5149) -> (-240.1481, 40.5189)
  line L4928 (-240.1481, 40.5189) -> (-239.7881, 40.5618)
  line L4929 (-239.7881, 40.5618) -> (-239.606, 40.6296)
  line L4930 (-239.606, 40.6296) -> (-239.4553, 40.7457)
  line L4931 (-239.4553, 40.7457) -> (-239.345, 40.9007)
  line L4932 (-239.345, 40.9007) -> (-239.2842, 41.0852)
  line L4933 (-239.2842, 41.0852) -> (-239.2635, 41.3297)
  line L4934 (-239.2635, 41.3297) -> (-239.2618, 41.5747)
  line L4935 (-239.2618, 41.5747) -> (-239.2792, 41.8191)
  line L4936 (-239.2792, 41.8191) -> (-239.3154, 42.0618)
  line L4937 (-239.3154, 42.0618) -> (-237.956, 42.2844)
  line L4938 (-237.956, 42.2844) -> (-237.8829, 41.8989)
  line L4939 (-237.8829, 41.8989) -> (-237.8389, 41.5095)
  line L4940 (-237.8389, 41.5095) -> (-237.8242, 41.1179)
  line L4941 (-237.8242, 41.1179) -> (-237.8389, 40.7258)
  line L4942 (-237.8389, 40.7258) -> (-237.8857, 40.3782)
  line L4943 (-237.8857, 40.3782) -> (-237.9657, 40.0938)
  line L4944 (-237.9657, 40.0938) -> (-238.0849, 39.8235)
  line L4945 (-238.0849, 39.8235) -> (-238.1832, 39.6674)
  line L4946 (-238.1832, 39.6674) -> (-238.2988, 39.5245)
  line L4947 (-238.2988, 39.5245) -> (-238.4306, 39.3964)
  line L4948 (-238.4306, 39.3964) -> (-238.5771, 39.2844)
  line L4949 (-238.5771, 39.2844) -> (-238.7803, 39.1711)
  line L4950 (-238.7803, 39.1711) -> (-239.2316, 39.0584)
  line L4951 (-239.2316, 39.0584) -> (-239.6943, 39.011)
  line L4952 (-239.6943, 39.011) -> (-240.1453, 38.9904)
  line L4953 (-240.1453, 38.9904) -> (-240.5967, 38.9836)
  line L4954 (-240.5967, 38.9836) -> (-245.8193, 38.9836)
  line L4955 (-245.8193, 38.9836) -> (-245.8193, 37.8586)
  line L4956 (-245.8193, 37.8586) -> (-247.0146, 37.8586)
  line L4957 (-247.0146, 37.8586) -> (-247.0146, 38.9836)
  line L4958 (-247.0146, 38.9836) -> (-249.2607, 38.9836)
  line L4959 (-249.2607, 38.9836) -> (-250.1865, 40.5149)
  line L4960 (-250.1865, 40.5149) -> (-247.0146, 40.5149)
  line L4961 (-247.2099, -5.2) -> (-247.1804, -4.9124)
  line L4962 (-247.1804, -4.9124) -> (-247.1233, -4.6297)
  line L4963 (-247.1233, -4.6297) -> (-247.0392, -4.3538)
  line L4964 (-247.0392, -4.3538) -> (-246.9287, -4.0867)
  line L4965 (-246.9287, -4.0867) -> (-246.678, -3.6839)
  line L4966 (-246.678, -3.6839) -> (-246.3519, -3.3462)
  line L4967 (-246.3519, -3.3462) -> (-245.9627, -3.0839)
  line L4968 (-245.9627, -3.0839) -> (-245.5224, -2.907)
  line L4969 (-245.5224, -2.907) -> (-245.1905, -2.823)
  line L4970 (-245.1905, -2.823) -> (-244.8536, -2.7649)
  line L4971 (-244.8536, -2.7649) -> (-244.5132, -2.7329)
  line L4972 (-244.5132, -2.7329) -> (-244.1709, -2.7273)
  line L4973 (-244.1709, -2.7273) -> (-237.9404, -2.7273)
  line L4974 (-237.9404, -2.7273) -> (-237.9404, -4.2546)
  line L4975 (-237.9404, -4.2546) -> (-243.6553, -4.2546)
  line L4976 (-243.6553, -4.2546) -> (-244.2042, -4.2718)
  line L4977 (-244.2042, -4.2718) -> (-244.749, -4.3406)
  line L4978 (-244.749, -4.3406) -> (-245.0166, -4.4176)
  line L4979 (-245.0166, -4.4176) -> (-245.2593, -4.5477)
  line L4980 (-245.2593, -4.5477) -> (-245.4696, -4.7256)
  line L4981 (-245.4696, -4.7256) -> (-245.6396, -4.9461)
  line L4982 (-245.6396, -4.9461) -> (-245.7262, -5.1021)
  line L4983 (-245.7262, -5.1021) -> (-245.7938, -5.2666)
  line L4984 (-245.7938, -5.2666) -> (-245.842, -5.4378)
  line L4985 (-245.842, -5.4378) -> (-245.8701, -5.614)
  line L4986 (-245.8701, -5.614) -> (-245.8837, -6.0642)
  line L4987 (-245.8837, -6.0642) -> (-245.8077, -6.5037)
  line L4988 (-245.8077, -6.5037) -> (-245.6457, -6.9192)
  line L4989 (-245.6457, -6.9192) -> (-245.4014, -7.2976)
  line L4990 (-245.4014, -7.2976) -> (-245.1943, -7.5109)
  line L4991 (-245.1943, -7.5109) -> (-244.9591, -7.6899)
  line L4992 (-244.9591, -7.6899) -> (-244.6999, -7.8319)
  line L4993 (-244.6999, -7.8319) -> (-244.4209, -7.9343)
  line L4994 (-244.4209, -7.9343) -> (-244.1242, -8.0073)
  line L4995 (-244.1242, -8.0073) -> (-243.8232, -8.0578)
  line L4996 (-243.8232, -8.0578) -> (-243.5194, -8.0856)
  line L4997 (-243.5194, -8.0856) -> (-243.2139, -8.0906)
  line L4998 (-243.2139, -8.0906) -> (-237.9404, -8.0906)
  line L4999 (-237.9404, -8.0906) -> (-237.9404, -9.6296)
  line L5000 (-237.9404, -9.6296) -> (-243.8349, -9.6296)
  line L5001 (-243.8349, -9.6296) -> (-244.1093, -9.634)
  line L5002 (-244.1093, -9.634) -> (-244.3819, -9.6603)
  line L5003 (-244.3819, -9.6603) -> (-244.6516, -9.7084)
  line L5004 (-244.6516, -9.7084) -> (-244.917, -9.7781)
  line L5005 (-244.917, -9.7781) -> (-245.1119, -9.8492)
  line L5006 (-245.1119, -9.8492) -> (-245.2928, -9.9484)
  line L5007 (-245.2928, -9.9484) -> (-245.4567, -10.0738)
  line L5008 (-245.4567, -10.0738) -> (-245.6006, -10.2234)
  line L5009 (-245.6006, -10.2234) -> (-245.7131, -10.409)
  line L5010 (-245.7131, -10.409) -> (-245.7976, -10.6077)
  line L5011 (-245.7976, -10.6077) -> (-245.8529, -10.8164)
  line L5012 (-245.8529, -10.8164) -> (-245.8779, -11.032)
  line L5013 (-245.8779, -11.032) -> (-245.8778, -11.4494)
  line L5014 (-245.8778, -11.4494) -> (-245.8037, -11.8601)
  line L5015 (-245.8037, -11.8601) -> (-245.694, -12.1577)
  line L5016 (-245.694, -12.1577) -> (-245.5459, -12.4382)
  line L5017 (-245.5459, -12.4382) -> (-245.3545, -12.6921)
  line L5018 (-245.3545, -12.6921) -> (-245.124, -12.9109)
  line L5019 (-245.124, -12.9109) -> (-244.8545, -13.0945)
  line L5020 (-244.8545, -13.0945) -> (-244.5882, -13.2141)
  line L5021 (-244.5882, -13.2141) -> (-244.3127, -13.309)
  line L5022 (-244.3127, -13.309) -> (-244.0298, -13.3787)
  line L5023 (-244.0298, -13.3787) -> (-243.7412, -13.4226)
  line L5024 (-243.7412, -13.4226) -> (-243.1953, -13.4717)
  line L5025 (-243.1953, -13.4717) -> (-242.6474, -13.4851)
  line L5026 (-242.6474, -13.4851) -> (-237.9404, -13.4851)
  line L5027 (-237.9404, -13.4851) -> (-237.9404, -15.0203)
  line L5028 (-237.9404, -15.0203) -> (-247.0146, -15.0203)
  line L5029 (-247.0146, -15.0203) -> (-247.0146, -13.6453)
  line L5030 (-247.0146, -13.6453) -> (-245.7412, -13.6453)
  line L5031 (-245.7412, -13.6453) -> (-246.0609, -13.4125)
  line L5032 (-246.0609, -13.4125) -> (-246.3485, -13.1433)
  line L5033 (-246.3485, -13.1433) -> (-246.6011, -12.8409)
  line L5034 (-246.6011, -12.8409) -> (-246.8154, -12.5086)
  line L5035 (-246.8154, -12.5086) -> (-246.9912, -12.1414)
  line L5036 (-246.9912, -12.1414) -> (-247.1201, -11.7507)
  line L5037 (-247.1201, -11.7507) -> (-247.1943, -11.3367)
  line L5038 (-247.1943, -11.3367) -> (-247.2217, -10.8953)
  line L5039 (-247.2217, -10.8953) -> (-247.2155, -10.6116)
  line L5040 (-247.2155, -10.6116) -> (-247.186, -10.3299)
  line L5041 (-247.186, -10.3299) -> (-247.1333, -10.0516)
  line L5042 (-247.1333, -10.0516) -> (-247.0576, -9.7781)
  line L5043 (-247.0576, -9.7781) -> (-246.9616, -9.5297)
  line L5044 (-246.9616, -9.5297) -> (-246.8383, -9.2968)
  line L5045 (-246.8383, -9.2968) -> (-246.6895, -9.0813)
  line L5046 (-246.6895, -9.0813) -> (-246.5173, -8.8852)
  line L5047 (-246.5173, -8.8852) -> (-246.3235, -8.7103)
  line L5048 (-246.3235, -8.7103) -> (-246.1101, -8.5586)
  line L5049 (-246.1101, -8.5586) -> (-245.8789, -8.4322)
  line L5050 (-245.8789, -8.4322) -> (-245.6318, -8.3328)
  line L5051 (-245.6318, -8.3328) -> (-245.994, -8.059)
  line L5052 (-245.994, -8.059) -> (-246.3271, -7.7507)
  line L5053 (-246.3271, -7.7507) -> (-246.6006, -7.4343)
  line L5054 (-246.6006, -7.4343) -> (-246.8232, -7.0906)
  line L5055 (-246.8232, -7.0906) -> (-246.9951, -6.7312)
  line L5056 (-246.9951, -6.7312) -> (-247.1201, -6.3523)
  line L5057 (-247.1201, -6.3523) -> (-247.1943, -5.95)
  line L5058 (-247.1943, -5.95) -> (-247.221, -5.5753)
  line L5059 (-247.221, -5.5753) -> (-247.2099, -5.2)
  line L5060 (-237.9404, 36.3977) -> (-237.9404, 34.8625)
  line L5061 (-237.9404, 34.8625) -> (-247.0146, 34.8625)
  line L5062 (-247.0146, 34.8625) -> (-247.0146, 36.3977)
  line L5063 (-247.0146, 36.3977) -> (-237.9404, 36.3977)
  line L5064 (-247.1904, 13.2024) -> (-247.0967, 13.593)
  line L5065 (-247.0967, 13.593) -> (-246.9404, 13.9914)
  line L5066 (-246.9404, 13.9914) -> (-246.7256, 14.3899)
  line L5067 (-246.7256, 14.3899) -> (-245.2959, 13.8625)
  line L5068 (-245.2959, 13.8625) -> (-245.4358, 13.599)
  line L5069 (-245.4358, 13.599) -> (-245.5391, 13.3205)
  line L5070 (-245.5391, 13.3205) -> (-245.6048, 13.0308)
  line L5071 (-245.6048, 13.0308) -> (-245.6318, 12.7336)
  line L5072 (-245.6318, 12.7336) -> (-245.5866, 12.3656)
  line L5073 (-245.5866, 12.3656) -> (-245.4549, 12.0247)
  line L5074 (-245.4549, 12.0247) -> (-245.2447, 11.7258)
  line L5075 (-245.2447, 11.7258) -> (-244.9639, 11.4836)
  line L5076 (-244.9639, 11.4836) -> (-244.7345, 11.3515)
  line L5077 (-244.7345, 11.3515) -> (-244.4873, 11.2571)
  line L5078 (-244.4873, 11.2571) -> (-244.0467, 11.1401)
  line L5079 (-244.0467, 11.1401) -> (-243.5989, 11.0579)
  line L5080 (-243.5989, 11.0579) -> (-243.1462, 11.0109)
  line L5081 (-243.1462, 11.0109) -> (-242.6904, 10.9993)
  line L5082 (-242.6904, 10.9993) -> (-237.9404, 10.9993)
  line L5083 (-237.9404, 10.9993) -> (-237.9404, 9.4602)
  line L5084 (-237.9404, 9.4602) -> (-247.0146, 9.4602)
  line L5085 (-247.0146, 9.4602) -> (-247.0146, 10.8469)
  line L5086 (-247.0146, 10.8469) -> (-245.6396, 10.8469)
  line L5087 (-245.6396, 10.8469) -> (-245.9281, 11.0051)
  line L5088 (-245.9281, 11.0051) -> (-246.2045, 11.1826)
  line L5089 (-246.2045, 11.1826) -> (-246.4681, 11.3788)
  line L5090 (-246.4681, 11.3788) -> (-246.7178, 11.593)
  line L5091 (-246.7178, 11.593) -> (-246.9328, 11.8556)
  line L5092 (-246.9328, 11.8556) -> (-247.091, 12.1522)
  line L5093 (-247.091, 12.1522) -> (-247.1885, 12.474)
  line L5094 (-247.1885, 12.474) -> (-247.2217, 12.8118)
  line L5095 (-247.2217, 12.8118) -> (-247.1904, 13.2024)
  line L5096 (-250.4639, -50.0554) -> (-250.4291, -49.217)
  line L5097 (-250.4291, -49.217) -> (-250.331, -48.3836)
  line L5098 (-250.331, -48.3836) -> (-250.2426, -47.9853)
  line L5099 (-250.2426, -47.9853) -> (-250.1184, -47.5993)
  line L5100 (-250.1184, -47.5993) -> (-249.9599, -47.2281)
  line L5101 (-249.9599, -47.2281) -> (-249.7683, -46.8736)
  line L5102 (-249.7683, -46.8736) -> (-249.545, -46.5382)
  line L5103 (-249.545, -46.5382) -> (-249.2913, -46.2241)
  line L5104 (-249.2913, -46.2241) -> (-249.0086, -45.9335)
  line L5105 (-249.0086, -45.9335) -> (-248.6982, -45.6687)
  line L5106 (-248.6982, -45.6687) -> (-248.2863, -45.3772)
  line L5107 (-248.2863, -45.3772) -> (-247.8502, -45.1254)
  line L5108 (-247.8502, -45.1254) -> (-247.3928, -44.9148)
  line L5109 (-247.3928, -44.9148) -> (-246.917, -44.7468)
  line L5110 (-246.917, -44.7468) -> (-246.2683, -44.5758)
  line L5111 (-246.2683, -44.5758) -> (-245.6093, -44.4554)
  line L5112 (-245.6093, -44.4554) -> (-244.9431, -44.386)
  line L5113 (-244.9431, -44.386) -> (-244.2724, -44.3679)
  line L5114 (-244.2724, -44.3679) -> (-243.5973, -44.3901)
  line L5115 (-243.5973, -44.3901) -> (-242.9248, -44.4539)
  line L5116 (-242.9248, -44.4539) -> (-242.3154, -44.5554)
  line L5117 (-242.3154, -44.5554) -> (-241.7591, -44.6986)
  line L5118 (-241.7591, -44.6986) -> (-241.2139, -44.8796)
  line L5119 (-241.2139, -44.8796) -> (-240.8743, -45.018)
  line L5120 (-240.8743, -45.018) -> (-240.5443, -45.1771)
  line L5121 (-240.5443, -45.1771) -> (-240.2249, -45.3564)
  line L5122 (-240.2249, -45.3564) -> (-239.917, -45.5554)
  line L5123 (-239.917, -45.5554) -> (-239.6696, -45.7432)
  line L5124 (-239.6696, -45.7432) -> (-239.435, -45.9462)
  line L5125 (-239.435, -45.9462) -> (-239.2138, -46.1638)
  line L5126 (-239.2138, -46.1638) -> (-239.0068, -46.3953)
  line L5127 (-239.0068, -46.3953) -> (-238.7753, -46.712)
  line L5128 (-238.7753, -46.712) -> (-238.575, -47.0483)
  line L5129 (-238.575, -47.0483) -> (-238.407, -47.4018)
  line L5130 (-238.407, -47.4018) -> (-238.2724, -47.7703)
  line L5131 (-238.2724, -47.7703) -> (-238.1478, -48.2327)
  line L5132 (-238.1478, -48.2327) -> (-238.0526, -48.7015)
  line L5133 (-238.0526, -48.7015) -> (-237.9874, -49.1755)
  line L5134 (-237.9874, -49.1755) -> (-237.9521, -49.6531)
  line L5135 (-237.9521, -49.6531) -> (-237.9404, -50.2039)
  line L5136 (-237.9404, -50.2039) -> (-237.9404, -54.7273)
  line L5137 (-237.9404, -54.7273) -> (-250.4678, -54.7273)
  line L5138 (-250.4678, -54.7273) -> (-250.4678, -50.4109)
  line L5139 (-250.4678, -50.4109) -> (-250.4639, -50.0554)
  line L5140 (-237.9404, -40.7742) -> (-237.9404, -42.3132)
  line L5141 (-237.9404, -42.3132) -> (-247.0146, -42.3132)
  line L5142 (-247.0146, -42.3132) -> (-247.0146, -40.7742)
  line L5143 (-247.0146, -40.7742) -> (-237.9404, -40.7742)
  line L5144 (-237.9404, -27.1687) -> (-237.9404, -28.7078)
  line L5145 (-237.9404, -28.7078) -> (-250.4678, -28.7078)
  line L5146 (-250.4678, -28.7078) -> (-250.4678, -27.1687)